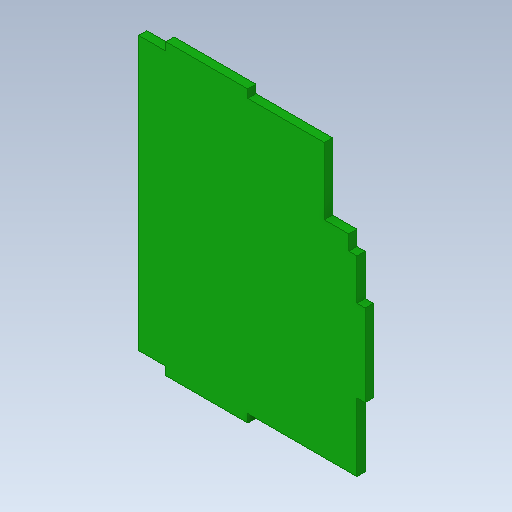
# Autodesk Inventor part: Celda pared divisora
Saved by Autodesk Inventor 2020 (Build 240168000, 168)
## iProperties
Created: 2020-03-12
Part Number: Celda pared divisora
Material: Genérico
Document SubType Name: Modeling
Designer: joser
Density: 1 g/cm^3
Appearance: Verde oscuro
Author: joser
Autodesk Inventor part; units mm, degrees
ref_plane "YZ Plane" through (0, 0, 0) normal (1, 0, 0) x (0, 1, 0)
ref_plane "XZ Plane" through (0, 0, 0) normal (0, 1, 0) x (-1, 0, 0)
ref_plane "XY Plane" through (0, 0, 0) normal (0, 0, 1) x (1, 0, 0)
sketch "Boceto1" plane through (0, 0, 0) normal (0, 0, 1) x (1, 0, 0)
  line L0 (0, 0) -> (0, 100)
  line L1 (80, 55) -> (83, 55)
  line L2 (83, 55) -> (83, 25)
  line L3 (83, 25) -> (80, 25)
  line L4 (80, 70) -> (80, 55)
  line L5 (80, 25) -> (80, 0)
  line L6 (10, 100) -> (10, 103)
  line L7 (10, 103) -> (40, 103)
  line L8 (40, 103) -> (40, 100)
  line L9 (0, 100) -> (10, 100)
  line L10 (40, 100) -> (68, 100)
  line L11 (77, 75.5) -> (68, 75.5)
  line L12 (68, 75.5) -> (68, 100)
  line L13 (10, 0) -> (10, -3)
  line L14 (40, -3) -> (40, 0)
  line L15 (10, -3) -> (40, -3)
  line L16 (80, 0) -> (40, 0)
  line L17 (10, 0) -> (0, 0)
  line L18 (80, 70) -> (77, 70)
  line L19 (77, 70) -> (77, 75.5)
  point P0 (0, 0)
  dimension "d5" = 30
  dimension "d9" = 30
  dimension "d11" = 10
  dimension "d13" = 3
  dimension "d16" = 80
  dimension "d17" = 3
  dimension "d22" = 3
  dimension "d23" = 100
  dimension "d24" = 25
  dimension "d26" = 3
  dimension "d29" = 9
  dimension "d30" = 70
  dimension "d31" = 75.5
  constraints: 40 end point, 14 perpendicular, 8 parallel, 5 collinear, 5 horizontal, 1 coincident, 1 vertical
  measures "d5" distance of L1.end L2.end
  measures "d9" distance of L6.end L7.end
  measures "d11" distance between parallel lines of L6 L0
  measures "d13" distance between parallel lines of L5 L2
  measures "d16" distance between parallel lines of L5 L0
  measures "d17" distance between parallel lines of L9 L7
  measures "d22" distance between parallel lines of L17 L15
  measures "d23" distance between parallel lines of L17 L9
  measures "d24" distance between parallel lines of L16 L3
  measures "d26" distance between parallel lines of L4 L19
  measures "d29" distance between parallel lines of L19 L12
  measures "d30" distance between parallel lines of L16 L18
  measures "d31" distance between parallel lines of L16 L11
extrude "Extrusión1" add sketch "Boceto1" along normal blind 3
